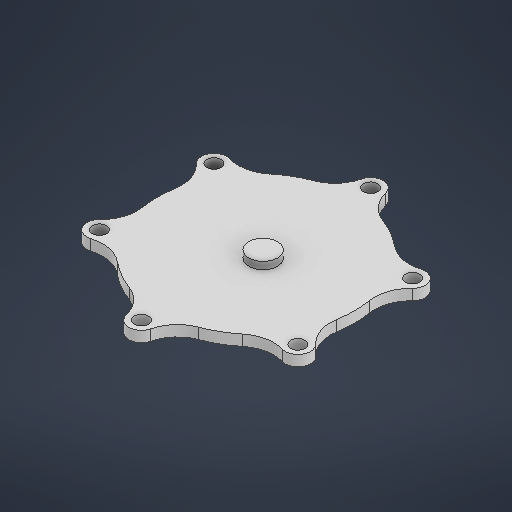
# Autodesk Inventor part: carcaza motor
Saved by Autodesk Inventor 2025.3 (Build 293356000, 356)
## iProperties
Created: 2025-10-02
Part Number: carcaza motor
Material: Generic
Document SubType Name: Modeling
Designer: sophi
Density: 1 g/cm^3
Appearance: Default
Author: sophi
Autodesk Inventor part; units mm, degrees
ref_plane "YZ Plane" through (0, 0, 0) normal (1, 0, 0) x (0, 1, 0)
ref_plane "XZ Plane" through (0, 0, 0) normal (0, 1, 0) x (-1, 0, 0)
ref_plane "XY Plane" through (0, 0, 0) normal (0, 0, 1) x (1, 0, 0)
sketch "Sketch1" plane through (0, 0, 0) normal (0, 1, 0) x (-1, 0, 0)
  circle A0 centre (0, 0) radius 27.5
  circle A1 centre (0, 0) radius 25
  circle A2 centre (0, -32) radius 3.5
  arc A3 (9.6311, -25.7583) -> (3.4049, -32.8102) centre (13.1333, -35.125) ccw
  line L0 (0, -39.6745) -> (0, -15.9391) construction
  arc A4 (-3.4049, -32.8102) -> (-9.6311, -25.7583) centre (-13.1333, -35.125) ccw
  line L1 (47.8103, 0) -> (-62.0389, 0) construction
  circle A5 centre (0, -32) radius 2
  circle A6 centre (27.7128, -16) radius 3.5
  circle A7 centre (27.7128, -16) radius 2
  arc A8 (26.712, -19.3539) -> (17.4918, -21.22) centre (23.8525, -28.9363) ccw
  arc A9 (27.1229, -4.5384) -> (30.1169, -13.4563) centre (36.9858, -6.1887) ccw
  circle A10 centre (27.7128, 16) radius 3.5
  circle A11 centre (27.7128, 16) radius 2
  arc A12 (30.1169, 13.4563) -> (27.1229, 4.5384) centre (36.9858, 6.1887) ccw
  arc A13 (17.4918, 21.22) -> (26.712, 19.3539) centre (23.8525, 28.9363) ccw
  circle A14 centre (0, 32) radius 3.5
  circle A15 centre (0, 32) radius 2
  arc A16 (3.4049, 32.8102) -> (9.6311, 25.7583) centre (13.1333, 35.125) ccw
  arc A17 (-9.6311, 25.7583) -> (-3.4049, 32.8102) centre (-13.1333, 35.125) ccw
  circle A18 centre (-27.7128, 16) radius 3.5
  circle A19 centre (-27.7128, 16) radius 2
  arc A20 (-26.712, 19.3539) -> (-17.4918, 21.22) centre (-23.8525, 28.9363) ccw
  arc A21 (-27.1229, 4.5384) -> (-30.1169, 13.4563) centre (-36.9858, 6.1887) ccw
  circle A22 centre (-27.7128, -16) radius 3.5
  circle A23 centre (-27.7128, -16) radius 2
  arc A24 (-30.1169, -13.4563) -> (-27.1229, -4.5384) centre (-36.9858, -6.1887) ccw
  arc A25 (-17.4918, -21.22) -> (-26.712, -19.3539) centre (-23.8525, -28.9363) ccw
  point P0 (27.1229, 4.5384)
  point P1 (30.1169, 13.4563)
  point P2 (17.4918, 21.22)
  point P3 (9.6311, 25.7583)
  point P4 (3.4049, 32.8102)
  point P5 (-17.4918, 21.22)
  point P6 (-26.712, 19.3539)
  point P7 (-27.1229, 4.5384)
  point P8 (-27.1229, -4.5384)
  point P9 (-30.1169, -13.4563)
  point P10 (-9.6311, -25.7583)
  point P11 (-3.4049, -32.8102)
  point P12 (26.712, -19.3539)
  point P13 (27.1229, -4.5384)
  dimension "d16" = 55
  dimension "d18" = 7
  dimension "d17" = 50
  dimension "d19" = 32
  dimension "d21" = 10
  dimension "d22" = 4
  dimension "d25" = 360
  constraints: 24 point on circle, 19 centre point, 8 coincident, 4 end point, 3 symmetric about line, 2 point on line, 1 horizontal, 1 vertical, 1 vertical alignment, 97 other
  measures "d17" diameter of A1
  measures "d19" distance of point (0, 0) point (0, -32)
  measures "d21" radius of A3
  measures "d22" diameter of A5
extrude "Extrusion5" add sketch "Sketch1" along normal blind 3
extrude "Extrusion6" add sketch "Sketch1" along normal blind 3 contours A1
sketch "Sketch8" plane through (0, 3, 0) normal (0, 1, 0) x (1, 0, 0)
  circle A0 centre (2, 0) radius 4
  circle A1 centre (2, 0) radius 22.5
  circle A2 centre (0, 0) radius 25 projected
  dimension "d50" = 8
  dimension "d51" = 45
  dimension "d52" = 2
  constraints: 2 centre point, 2 horizontal alignment, 1 concentric
  measures "d50" diameter of A0
  measures "d51" diameter of A1
  measures "d52" distance of A1.centre A2.centre
extrude "Extrusion11" add sketch "Sketch8" along normal blind 2 contours A0
body "Solid2"
